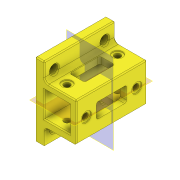
# Autodesk Inventor part: Part3
Saved by Autodesk Inventor 2021 (Build 250183000, 183)
## iProperties
Created: 2021-02-20
Part Number: Part3
Material: Generic
Document SubType Name: Modeling
Designer: dsdan
Density: 1 g/cm^3
Appearance: Default
Author: dsdan
Autodesk Inventor part; units mm, degrees
ref_plane "YZ Plane" through (0, 0, 0) normal (1, 0, 0) x (0, 1, 0)
ref_plane "XZ Plane" through (0, 0, 0) normal (0, 1, 0) x (-1, 0, 0)
ref_plane "XY Plane" through (0, 0, 0) normal (0, 0, 1) x (1, 0, 0)
sketch "Sketch1" plane through (0, 0, 0) normal (0, 0, 1) x (1, 0, 0)
  line L0 (-21.4968, -52.8892) -> (-21.4968, 25.0724)
  circle A0 centre (0, -16.4084) radius 3 construction
  arc A1 (-5.4102, -9.5755) -> (5.4102, -9.5755) centre (0, 0) ccw construction
  line L1 (-5.4102, -9.5755) -> (-5.4102, -5.6134) construction
  line L2 (-5.4102, -5.6134) -> (-3.7592, -5.6134) construction
  line L3 (-3.7592, -5.6134) -> (-3.2512, -5.1054) construction
  line L4 (-3.2512, -5.1054) -> (-3.2512, -3.9116) construction
  line L5 (-3.2512, -3.9116) -> (-11.4808, -3.9116) construction
  line L6 (-11.4808, -3.9116) -> (-12.4968, -4.9276) construction
  line L7 (-12.4968, -4.9276) -> (-12.4968, -13.1572) construction
  line L8 (-12.4968, -13.1572) -> (-11.303, -13.1572) construction
  line L9 (-11.303, -13.1572) -> (-10.795, -12.6492) construction
  line L10 (-10.795, -12.6492) -> (-10.795, -11.0109) construction
  line L11 (-10.795, -11.0109) -> (-6.8257, -11.0109) construction
  arc A2 (-6.8257, -21.8059) -> (-6.8257, -11.0109) centre (-16.4084, -16.4084) ccw construction
  line L12 (-6.8257, -21.8059) -> (-10.795, -21.8059) construction
  line L13 (-10.795, -21.8059) -> (-10.795, -20.1676) construction
  line L14 (-10.795, -20.1676) -> (-11.303, -19.6596) construction
  line L15 (-11.303, -19.6596) -> (-12.4968, -19.6596) construction
  line L16 (-12.4968, -19.6596) -> (-12.4968, -27.8892) construction
  line L17 (-12.4968, -27.8892) -> (-11.4808, -28.9052) construction
  line L18 (-11.4808, -28.9052) -> (-3.2512, -28.9052) construction
  line L19 (-3.2512, -28.9052) -> (-3.2512, -27.7114) construction
  line L20 (-3.2512, -27.7114) -> (-3.7592, -27.2034) construction
  line L21 (-3.7592, -27.2034) -> (-5.4102, -27.2034) construction
  line L22 (-5.4102, -27.2034) -> (-5.4102, -23.2413) construction
  arc A3 (5.4102, -23.2413) -> (-5.4102, -23.2413) centre (0, -32.8168) ccw construction
  line L23 (5.4102, -23.2413) -> (5.4102, -27.2034) construction
  line L24 (5.4102, -27.2034) -> (3.7592, -27.2034) construction
  line L25 (3.7592, -27.2034) -> (3.2512, -27.7114) construction
  line L26 (3.2512, -27.7114) -> (3.2512, -28.9052) construction
  line L27 (3.2512, -28.9052) -> (11.4808, -28.9052) construction
  line L28 (11.4808, -28.9052) -> (12.4968, -27.8892) construction
  line L29 (12.4968, -27.8892) -> (12.4968, -19.6596) construction
  line L30 (12.4968, -19.6596) -> (11.303, -19.6596) construction
  line L31 (11.303, -19.6596) -> (10.795, -20.1676) construction
  line L32 (10.795, -20.1676) -> (10.795, -21.8059) construction
  line L33 (10.795, -21.8059) -> (6.8257, -21.8059) construction
  arc A4 (6.8257, -11.0109) -> (6.8257, -21.8059) centre (16.4084, -16.4084) ccw construction
  line L34 (6.8257, -11.0109) -> (10.795, -11.0109) construction
  line L35 (10.795, -11.0109) -> (10.795, -12.6492) construction
  line L36 (10.795, -12.6492) -> (11.303, -13.1572) construction
  line L37 (11.303, -13.1572) -> (12.4968, -13.1572) construction
  line L38 (12.4968, -13.1572) -> (12.4968, -4.9276) construction
  line L39 (12.4968, -4.9276) -> (11.4808, -3.9116) construction
  line L40 (11.4808, -3.9116) -> (3.2512, -3.9116) construction
  line L41 (3.2512, -3.9116) -> (3.2512, -5.1054) construction
  line L42 (3.2512, -5.1054) -> (3.7592, -5.6134) construction
  line L43 (3.7592, -5.6134) -> (5.4102, -5.6134) construction
  line L44 (5.4102, -5.6134) -> (5.4102, -9.5755) construction
  circle A5 centre (-8.4963, -7.9121) radius 2.0193 construction
  circle A6 centre (8.4963, -24.9047) radius 2.0193 construction
  circle A7 centre (0, -16.4084) radius 3 construction
  circle A8 centre (-8.4963, -24.9047) radius 2.0193 construction
  circle A9 centre (8.4963, -7.9121) radius 2.0193 construction
  line L45 (-21.4968, -52.8892) -> (-12.4968, -52.8892)
  line L46 (-12.4968, -52.8892) -> (-12.4968, -39.4052)
  line L47 (-12.4968, 6.5884) -> (-12.4968, 20.0724)
  line L48 (-12.4968, 20.0724) -> (-21.4968, 20.0724)
  line L49 (-12.4968, -19.6596) -> (-12.4968, -13.1572) construction
  line L50 (-8.4968, -35.4052) -> (18.9968, -35.4052)
  line L51 (18.9968, 2.5884) -> (-8.4968, 2.5884)
  line L52 (3.2512, -28.9052) -> (-3.2512, -28.9052) construction
  line L53 (3.2512, -3.9116) -> (-3.2512, -3.9116) construction
  arc A10 (-8.4968, -35.4052) -> (-12.4968, -39.4052) centre (-8.4968, -39.4052) ccw
  arc A11 (-12.4968, 6.5884) -> (-8.4968, 2.5884) centre (-8.4968, 6.5884) ccw
  line L54 (18.9968, -35.4052) -> (18.9968, 2.5884)
  line L55 (11.4808, -28.9052) -> (12.4968, -28.9052) construction
  line L56 (12.4968, -28.9052) -> (12.4968, -3.9116) construction
  line L57 (12.4968, -3.9116) -> (11.4808, -3.9116) construction
  line L58 (-12.5468, -3.8616) -> (-12.5468, -28.9552)
  line L59 (-12.5468, -28.9552) -> (12.5468, -28.9552)
  line L60 (12.5468, -28.9552) -> (12.5468, -3.8616)
  line L61 (12.5468, -3.8616) -> (-12.5468, -3.8616)
  line L62 (-12.5468, -3.8616) -> (12.5468, -28.9552) construction
  line L63 (-12.5468, -28.9552) -> (12.5468, -3.8616) construction
  dimension "d0" = 25
  dimension "d1" = 25
  dimension "d3" = 6.5
  dimension "d4" = 6.5
  dimension "d6" = 4
  dimension "d30" = 6.5
  dimension "d45" = 9
  dimension "d61" = 0.05
  dimension "d62" = 0.05
  constraints: 41 end point, 6 perpendicular, 5 point on line, 4 point on circle, 4 tangent, 3 collinear, 3 horizontal, 3 parallel, 2 centre point, 2 midpoint, 2 vertical, 1 equal radius
  measures "d0" distance of L6.end L47.end
  measures "d1" distance of L45.end L16.end
  measures "d3" distance between parallel lines of L27 L50
  measures "d4" vertical distance of L39.end L51.start
  measures "d6" radius of A10
  measures "d30" distance between parallel lines of L29 L54
  measures "d45" distance between parallel lines of L47 L0
  measures "d61" distance between parallel lines of L29 L60
  measures "d62" distance between parallel lines of L18 L59
extrude "Extrusion1" add sketch "Sketch1" against normal blind 70
sketch "Sketch2" plane through (18.9968, 2.5884, 0) normal (1, 0, 0) x (0, -1, 0)
  circle A0 centre (18.9968, 60) radius 5.1
  line L0 (37.9936, 0) -> (37.9936, 70) construction
  line L1 (0, 0) -> (37.9936, 70) construction
  line L2 (37.9936, 0) -> (0, 70) construction
  point P0 (18.9968, 35)
  point P1 (18.9968, 35)
  dimension "d9" = 10.2
  dimension "d54" = 25
  constraints: 4 end point, 2 midpoint, 1 centre point, 1 coincident, 1 vertical alignment
  measures "d9" diameter of A0
  measures "d54" distance of A0.centre point (18.997, 35)
extrude "Extrusion2" cut sketch "Sketch2" against normal blind 1
sketch "Sketch3" plane through (17.9968, -16.4084, -60) normal (1, 0, 0) x (0, 0, -1)
  circle A0 centre (0, 0) radius 3.05
  circle A1 centre (0, 0) radius 5.1 projected
  point P0 (-60, 16.4084)
  point P1 (4.9808, -1.0962)
  dimension "d14" = 6.1
  constraints: 1 centre point, 2 other
  measures "d14" diameter of A0
extrude "Extrusion3" cut sketch "Sketch3" against normal blind 10 contours A0
sketch "Sketch4" plane through (-21.4968, -52.8892, 0) normal (-1, 0, 0) x (0, 0, 1)
  line L0 (0, 72.9616) -> (0, 0) projected
  line L1 (0, 0) -> (-70, 0) projected
  line L2 (-70, 0) -> (-70, 72.9616) projected
  circle A0 centre (-10, 11.4808) radius 3.05
  line L3 (0, 72.9616) -> (-70, 72.9616) projected
  line L4 (0, 0) -> (-70, 0) projected
  line L5 (-35, 0) -> (-35, 72.9616) construction
  line L6 (-70, 36.4808) -> (0, 36.4808) construction
  circle A1 centre (-60, 11.4808) radius 3.05
  circle A2 centre (-10, 61.4808) radius 3.05
  circle A3 centre (-60, 61.4808) radius 3.05
  point P0 (0, 52.8892)
  dimension "d21" = 6.1
  dimension "d35" = 25
  dimension "d36" = 25
  dimension "d39" = 50
  dimension "d42" = 50
  constraints: 4 centre point, 4 end point, 4 midpoint, 1 horizontal, 1 vertical, 6 other
  measures "d21" diameter of A0
  measures "d35" distance from line of L5 A0.centre
  measures "d36" distance from line of L6 A0.centre
  measures "d39" distance of A0.centre A1.centre
  measures "d42" distance of A0.centre A2.centre
extrude "Extrusion4" cut sketch "Sketch4" against normal through all contours A0 | A1 | A2 | A3
sketch "Sketch6" plane through (-12.4968, 6.5884, -12.2999) normal (1, 0, 0) x (0, 0, -1)
  circle A0 centre (47.7001, 2.0032) radius 3.05 projected
  circle A1 centre (47.7001, 2.0032) radius 4
  circle A2 centre (-2.2999, 2.0032) radius 3.05 projected
  circle A3 centre (-2.2999, 2.0032) radius 4
  circle A4 centre (-2.2999, -47.9968) radius 3.05 projected
  circle A5 centre (-2.2999, -47.9968) radius 4
  arc A6 (45.4001, -45.9936) -> (50, -45.9936) centre (47.7001, -47.9968) ccw projected
  circle A7 centre (47.7001, -47.9968) radius 4
  point P0 (-12.2999, -6.5884)
  dimension "d46" = 8
  dimension "d47" = 8
  dimension "d48" = 8
  dimension "d49" = 8
  constraints: 4 centre point, 4 coincident
  measures "d46" diameter of A1
  measures "d47" diameter of A3
  measures "d48" diameter of A5
  measures "d49" diameter of A7
extrude "Extrusion6" cut sketch "Sketch6" along normal blind 5 and the other way blind 6 contours A0 | A1 | A2 | A3 | A4 | A5 | A7
ref_plane "Work Plane2" through (0, 0, -35) normal (0, 0, -1) x (-1, 0, 0)
mirror "Mirror2" about plane through (0, 0, -35) normal (0, 0, -1) of "Extrusion2", "Extrusion3"
sketch "Sketch9" plane through (18.9968, -35.4052, 0) normal (1, 0, 0) x (0, 0, -1)
  line L0 (22, 11.4968) -> (48, 11.4968)
  line L1 (50, 13.4968) -> (50, 24.4968)
  line L2 (48, 26.4968) -> (22, 26.4968)
  line L3 (20, 24.4968) -> (20, 13.4968)
  line L4 (20, 11.4968) -> (50, 26.4968) construction
  line L5 (50, 11.4968) -> (20, 26.4968) construction
  circle A0 centre (60, 18.9968) radius 3.05 projected
  circle A1 centre (10, 18.9968) radius 5.1 projected
  circle A2 centre (60, 18.9968) radius 5.1 projected
  line L6 (0, 0) -> (0, 37.9936) projected
  line L7 (0, 0) -> (70, 0) projected
  line L8 (70, 37.9936) -> (70, 0) projected
  line L9 (0, 37.9936) -> (70, 37.9936) projected
  arc A3 (50, 24.4968) -> (48, 26.4968) centre (48, 24.4968) ccw
  arc A4 (48, 11.4968) -> (50, 13.4968) centre (48, 13.4968) ccw
  arc A5 (20, 13.4968) -> (22, 11.4968) centre (22, 13.4968) ccw
  arc A6 (22, 26.4968) -> (20, 24.4968) centre (22, 24.4968) ccw
  point P0 (0, 35.4052)
  point P1 (35, 18.9968)
  point P2 (35, 18.9968)
  point P3 (35, 18.9968)
  point P4 (35, 37.9936)
  dimension "d55" = 15
  dimension "d56" = 30
  dimension "d57" = 2
  dimension "d58" = 2
  constraints: 12 end point, 8 point on circle, 8 point on line, 8 tangent, 5 midpoint, 4 centre point, 2 equal radius, 2 parallel, 1 horizontal, 1 horizontal alignment, 1 perpendicular, 1 vertical alignment
  measures "d55" distance between parallel lines of L2 L0
  measures "d56" distance of L4.start L5.start
  measures "d57" radius of A3
  measures "d58" radius of A6
extrude "Extrusion7" cut sketch "Sketch9" against normal up to surface (31.5436 mm away) contours A5 L3 A6 L2 A3 L1 A4 L0
chamfer "Chamfer1" distance 1 angle 45 23 edges at (-12.4968, 20.0724, -35) (-21.4968, 20.0724, -35) (-12.4968, -52.8892, -35) (-21.4968, -52.8892, -35) (-11.3252, 3.76, 0) (-12.4968, 13.3304, 0) (5.25, 2.5884, 0) (-16.9968, 20.0724, 0) (-16.9968, 20.0724, -70) (-21.4968, -16.4084, 0) (-21.4968, -16.4084, -70) (-12.4968, 13.3304, -70) (-11.3252, 3.76, -70) (5.25, 2.5884, -70) (5.25, -35.4052, -70) (-11.3252, -36.5768, -70) (-12.4968, -46.1472, -70) (-16.9968, -52.8892, -70) (-16.9968, -52.8892, 0) (18.9968, 2.5884, -35) (18.9968, -16.4084, -70) (18.9968, -35.4052, -35) (18.9968, -16.4084, 0)
chamfer "Chamfer2" distance 1 angle 45 12 edges at (-11.9627, 4.5916, -9.9964) (-12.4968, 7.5545, -13.8632) (-12.4968, 12.4548, -8.9629) (-11.9627, 4.5916, -59.9964) (-12.4968, 7.5545, -63.8632) (-12.4968, 12.4548, -58.9629) (-12.4968, -45.2716, -8.9629) (-12.4968, -40.3713, -13.8632) (-11.9627, -37.4084, -10.0036) (-12.4968, -40.3713, -63.8632) (-12.4968, -45.2716, -58.9629) (-11.9627, -37.4084, -60.0036)
sketch "Sketch10" plane through (-8.4968, 2.5884, -1) normal (0, 1, 0) x (1, 0, 0)
  circle A0 centre (8.4968, 9) radius 3.05
  circle A1 centre (8.4968, 59) radius 3.05
  line L0 (-4.05, -1) -> (21.0436, -1) projected
  line L1 (21.0436, 69) -> (-4.05, 69) projected
  line L2 (26.4936, 12.05) -> (26.4936, 5.95) projected
  line L3 (26.4936, 62.05) -> (26.4936, 55.95) projected
  point P0 (8.4968, -1)
  point P1 (8.4968, -1)
  point P2 (26.4936, 9)
  point P3 (26.4936, 59)
  dimension "d67" = 6.1
  constraints: 3 midpoint, 2 centre point, 2 horizontal alignment, 2 vertical alignment, 1 equal radius
  measures "d67" diameter of A1
extrude "Extrusion8" cut sketch "Sketch10" against normal through all
sketch "Sketch11" plane through (-8.4968, 2.5884, -1) normal (0, 1, 0) x (1, 0, 0)
  circle A0 centre (8.4968, 9) radius 3.05 projected
  circle A1 centre (8.4968, 9) radius 5.1
  circle A2 centre (8.4968, 59) radius 3.05 projected
  circle A3 centre (8.4968, 59) radius 5.1
  point P0 (8.4968, -1)
  dimension "d70" = 10.2
  dimension "d71" = 10.2
  constraints: 2 centre point, 2 coincident
  measures "d70" diameter of A1
  measures "d71" diameter of A3
extrude "Extrusion9" cut sketch "Sketch11" against normal blind 1
ref_plane "Work Plane3" through (-8.4968, -16.4084, -1) normal (0, 1, 0) x (1, 0, 0)
mirror "Mirror3" about plane through (-8.4968, -16.4084, -1) normal (0, 1, 0) of "Extrusion9"
chamfer "Chamfer3" distance 1 angle 45 8 edges at (0, -3.8616, 0) (12.5468, -16.4084, 0) (0, -28.9552, 0) (-12.5468, -16.4084, 0) (-12.5468, -16.4084, -70) (0, -28.9552, -70) (12.5468, -16.4084, -70) (0, -3.8616, -70)
sketch "Sketch12" plane through (-8.4968, 2.5884, -1) normal (0, 1, 0) x (1, 0, 0)
  line L0 (2.9968, 19) -> (13.9968, 19)
  line L1 (15.9968, 21) -> (15.9968, 47)
  line L2 (13.9968, 49) -> (2.9968, 49)
  line L3 (0.9968, 47) -> (0.9968, 21)
  line L4 (0.9968, 19) -> (15.9968, 49) construction
  line L5 (15.9968, 19) -> (0.9968, 49) construction
  arc A0 (15.9968, 47) -> (13.9968, 49) centre (13.9968, 47) ccw
  arc A1 (13.9968, 19) -> (15.9968, 21) centre (13.9968, 21) ccw
  arc A2 (0.9968, 21) -> (2.9968, 19) centre (2.9968, 21) ccw
  arc A3 (2.9968, 49) -> (0.9968, 47) centre (2.9968, 47) ccw
  circle A4 centre (8.4968, 9) radius 3.05 projected
  circle A5 centre (8.4968, 59) radius 3.05 projected
  point P0 (8.4968, -1)
  point P1 (8.4968, 34)
  point P2 (8.4968, 34)
  point P3 (8.4968, 34)
  dimension "d77" = 30
  dimension "d78" = 15
  dimension "d79" = 2
  dimension "d80" = 2
  dimension "d81" = 25
  dimension "d82" = 25
  constraints: 12 end point, 8 point on circle, 8 point on line, 8 tangent, 4 centre point, 4 midpoint, 2 equal radius, 2 parallel, 1 horizontal, 1 perpendicular, 1 vertical alignment
  measures "d77" distance between parallel lines of L2 L0
  measures "d78" distance of L4.start L5.start
  measures "d79" radius of A0
  measures "d80" radius of A3
  measures "d81" distance of point (8.497, 34) A4.centre
  measures "d82" distance of A5.centre point (8.497, 34)
extrude "Extrusion10" cut sketch "Sketch12" against normal through all contours A2 L3 A3 L2 A0 L1 A1 L0
equation "\"d1\" = d0"
equation "\"d81\" = d82"
body "Solid1"
